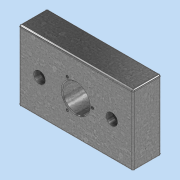
# Autodesk Inventor part: Oben
Saved by Autodesk Inventor 2021 (Build 250183000, 183)
## iProperties
Created: 2024-03-13
Part Number: Oben
Material: Generic
Document SubType Name: Modeling
Designer: Nokia
Density: 1 g/cm^3
Appearance: Steel Galvanized
Mass: 2523.72 g
Surface Area: 1483.16 cm^2
Volume: 2523.72 cm^3
Author: Nokia
Autodesk Inventor part; units mm, degrees
ref_plane "YZ Plane" through (0, 0, 0) normal (1, 0, 0) x (0, 1, 0)
ref_plane "XZ Plane" through (0, 0, 0) normal (0, 1, 0) x (-1, 0, 0)
ref_plane "XY Plane" through (0, 0, 0) normal (0, 0, 1) x (1, 0, 0)
sketch "Sketch1" plane through (0, 0, 0) normal (0, 0, 1) x (1, 0, 0)
  line L0 (130, -80) -> (130, 80)
  line L1 (130, 80) -> (-130, 80)
  line L2 (-130, 80) -> (-130, -80)
  line L3 (-130, -80) -> (130, -80)
  point P0 (0, 0)
  dimension "d2" = 260
  dimension "d3" = 160
  constraints: 8 end point, 3 perpendicular
  measures "d2" distance of L0.end L1.end
  measures "d3" distance of L1.end L2.end
extrude "Extrusion1" add sketch "Sketch1" along normal blind 65
sketch "Sketch2" plane through (0, 0, 65) normal (0, 0, 1) x (1, 0, 0)
  circle A0 centre (0, 0) radius 31
  circle A1 centre (0, 0) radius 19
  circle A2 centre (0, 0) radius 38
  circle A3 centre (38, 0.0213) radius 3.5
  dimension "d12" = 76
  dimension "d6" = 62
  dimension "d9" = 38
  dimension "d13" = 7
  constraints: 3 centre point, 3 coincident, 3 other
  measures "d6" diameter of A0
  measures "d9" diameter of A1
  measures "d13" diameter of A3
extrude "Extrusion2" cut sketch "Sketch2" against normal blind 56 contours A0 | A1
extrude "Extrusion3" cut sketch "Sketch2" against normal through all contours A1
hole "Hole1" at (38, 0.0213, 65) direction (0, 0, -1) diameter 4.917 depth 46 tip angle 118 thread size "M6x1" class "6H" standard "ISO Metric profile"
pattern_circular "Circular Pattern1" count 3 over 360 about axis through (0, 0, -10) along (0, 0, 1) of "Hole1"
sketch "Sketch3" plane through (0, 0, 0) normal (0, 0, -1) x (-1, 0, 0)
  line L0 (130, 80) -> (130, -80) projected
  circle A0 centre (0, 0) radius 19 projected
  circle A1 centre (82, 0) radius 13
  circle A2 centre (-82, 0) radius 13
  line L1 (-130, -80) -> (-130, 80) projected
  dimension "d25" = 26
  dimension "d26" = 48
  dimension "d27" = 48
  constraints: 2 centre point
  measures "d25" diameter of A1
  measures "d26" distance from line of L0 A1.centre
  measures "d27" distance from line of L1 A2.centre
extrude "Extrusion4" cut sketch "Sketch3" against normal blind 45 contours A1 | A2
sketch "Sketch4" plane through (0, 0, 65) normal (0, 0, 1) x (1, 0, 0)
  circle A0 centre (82, 0) radius 13 projected
  circle A1 centre (82, 0) radius 13
  circle A2 centre (-82, 0) radius 13 projected
  circle A3 centre (-82, 0) radius 13
  point P0 (0, 0)
  constraints: 2 centre point, 2 coincident
extrude "Extrusion5" cut sketch "Sketch4" against normal blind 15
sketch "Sketch5" plane through (82, 0, 50) normal (0, 0, 1) x (1, 0, 0)
  circle A0 centre (6.5, 0) radius 3.5
  line L0 (-82, 0) -> (-82, 25.4786)
  circle A1 centre (-3.25, 5.6292) radius 3.5
  circle A2 centre (-3.25, -5.6292) radius 3.5
  circle A3 centre (-170.5, 0) radius 3.5
  circle A4 centre (-160.75, 5.6292) radius 3.5
  circle A5 centre (-160.75, -5.6292) radius 3.5
  point P0 (0, 0)
  dimension "d33" = 7
  dimension "d36" = 360
  dimension "d45" = 6.5
  constraints: 6 centre point, 3 symmetric about line, 2 end point, 1 coincident, 1 vertical, 10 other
  measures "d33" diameter of A0
  measures "d45" distance of point (6.5, 0) point (0, 0)
hole "Hole2" at (-88.5, 0, 50) at (-78.75, 5.6292, 50) at (-78.75, -5.6292, 50) at (78.75, -5.6292, 50) at (88.5, 0, 50) at (78.75, 5.6292, 50) direction (0, 0, -1) diameter 6 end through all
sketch "Sketch7" plane through (-130, -80, 0) normal (0, -1, 0) x (1, 0, 0)
  line L0 (260, 65) -> (0, 65)
  line L1 (260, 65) -> (260, 0)
  line L2 (260, 0) -> (0, 0)
  line L3 (0, 32.5) -> (0, 65)
  line L4 (0, 65) -> (260, 65)
  line L5 (0, 32.5) -> (260, 32.5)
  line L6 (130, 48.75) -> (195, 48.75)
  line L7 (130, 65) -> (130, 0)
  line L8 (195, 65) -> (195, 0)
  line L9 (162.5, 65) -> (162.5, 0)
  circle A0 centre (162.5, 48.75) radius 7
  circle A1 centre (227.5, 48.75) radius 7
  circle A2 centre (227.5, 16.25) radius 7
  circle A3 centre (162.5, 16.25) radius 7
  circle A4 centre (32.5, 16.25) radius 7
  circle A5 centre (32.5, 48.75) radius 7
  circle A6 centre (97.5, 48.75) radius 7
  circle A7 centre (97.5, 16.25) radius 7
  circle A8 centre (162.5, 48.75) radius 14
  circle A9 centre (227.5, 48.75) radius 14
  circle A10 centre (227.5, 16.25) radius 14
  circle A11 centre (162.5, 16.25) radius 14
  circle A12 centre (32.5, 48.75) radius 14
  circle A13 centre (32.5, 16.25) radius 14
  circle A14 centre (97.5, 16.25) radius 14
  circle A15 centre (97.5, 48.75) radius 14
  line L10 (260, 0) -> (0, 0) projected
  dimension "d64" = 65
  dimension "d65" = 14
  dimension "d66" = 28
  dimension "d67" = 0
  dimension "d68" = 0
  constraints: 20 end point, 16 centre point, 14 symmetric about line, 7 point on line, 6 perpendicular, 3 midpoint, 2 coincident, 1 vertical, 15 other
  measures "d64" distance of L4.end L1.end
  measures "d65" diameter of A0
  measures "d66" diameter of A8
  measures "d67" distance of point (0, 0) L2.end
  measures "d68" distance of point (0, 0) L2.end
hole "Hole5" at (-97.5, -80, 48.75) at (-97.5, -80, 16.25) at (-32.5, -80, 16.25) at (-32.5, -80, 48.75) at (32.5, -80, 16.25) at (32.5, -80, 48.75) at (97.5, -80, 16.25) at (97.5, -80, 48.75) direction (0, 1, 0) diameter 10.106 depth 65 tip angle 118 thread size "M12x1.75" class "6H" standard "ISO Metric profile"
fillet "Fillet1" radius 4 12 edges at (130, 0, 65) (130, 0, 0) (0, -80, 0) (0, -80, 65) (-130, 0, 65) (-130, 0, 0) (0, 80, 65) (0, 80, 0) (130, 80, 32.5) (130, -80, 32.5) (-130, -80, 32.5) (-130, 80, 32.5)
chamfer "Chamfer1" distance 1 angle 45 8 edges at (97.5, -80, 53.803) (97.5, -80, 21.303) (32.5, -80, 53.803) (32.5, -80, 21.303) (-32.5, -80, 53.803) (-32.5, -80, 21.303) (-97.5, -80, 53.803) (-97.5, -80, 21.303)
chamfer "Chamfer2" distance 2 angle 45 3 edges at (95, 0, 0) (-69, 0, 0) (-31, 0, 65)
chamfer "Chamfer3" distance 0.5 angle 45 3 edges at (-21.1476, 31.6691, 65) (38, 2.4798, 65) (-16.8524, -34.1489, 65)
body "Solid1"
